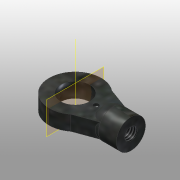
# Autodesk Inventor part: 500-103
Saved by Autodesk Inventor 2016 (Build 200138000, 138)
## iProperties
Created: 2015-04-18
Part Number: 500-103
Material: Steel
Document SubType Name: Modeling
Designer: Station9
Density: 7.85 g/cm^3
Appearance: Plate
Mass: 2.13897 g
Surface Area: 4.39252 cm^2
Volume: 0.27248 cm^3
Author: Station9
Autodesk Inventor part; units mm, degrees
ref_plane "YZ Plane" through (0, 0, 0) normal (1, 0, 0) x (0, 1, 0)
ref_plane "XZ Plane" through (0, 0, 0) normal (0, 1, 0) x (-1, 0, 0)
ref_plane "XY Plane" through (0, 0, 0) normal (0, 0, 1) x (1, 0, 0)
sketch "Sketch1" plane through (0, 0, 0) normal (0, 1, 0) x (-1, 0, 0)
  line L0 (3.5, 0) -> (-5.6696, 0) construction
  line L1 (0, -2.85) -> (3.5, -2.85)
  arc A0 (3.5, -2.85) -> (6.35, 0) centre (3.5, 0) ccw
  line L2 (0, 0) -> (0, -2.85)
  line L3 (0, 0) -> (6.35, 0)
  point P0 (-1.0848, 0)
  dimension "d0" = 2.85
  dimension "d1" = 3.5
  constraints: 10 end point, 2 point on circle, 1 centre point, 1 horizontal, 1 midpoint, 1 perpendicular, 1 tangent
  measures "d0" radius of A0
  measures "d1" distance from line of L2 L0.start
revolve "Revolution1" add sketch "Sketch1" angle 360 about axis through (-3.5, 0, 0) along (1, 0, 0)
sketch "Sketch2" plane through (0, 0, 0) normal (0, 0, 1) x (1, 0, 0)
  arc A0 (-7.7327, 3.9972) -> (-7.7396, -4.0028) centre (-10.9, 0) ccw
  line L0 (0, -2.85) -> (0, 2.85) projected
  line L1 (-3.5, -2.4597) -> (-7.7396, -4.0028)
  line L2 (-3.5, 2.4567) -> (-7.7327, 3.9972)
  arc A1 (-3.5, 2.85) -> (-6.35, 0) centre (-3.5, 0) ccw projected
  line L3 (-3.5, 2.85) -> (0, 2.85) projected
  line L4 (0, 2.85) -> (0, -2.85) projected
  line L5 (0, -2.85) -> (-3.5, -2.85) projected
  arc A2 (-6.35, 0) -> (-3.5, -2.85) centre (-3.5, 0) ccw projected
  line L6 (-3.5, 2.4567) -> (-3.5, -2.4597)
  line L7 (-3.5, -2.85) -> (-3.5, 2.85) projected
  point P0 (0, 0)
  dimension "d3" = 10.2
  dimension "d4" = 10.9
  dimension "d7" = 8
  dimension "d12" = 110
  dimension "d13" = 110
  constraints: 6 end point, 2 point on circle, 2 vertical alignment, 1 centre point, 1 collinear
  measures "d3" diameter of A0
  measures "d4" distance from line of L0 A0.centre
  measures "d7" distance of L1.end L2.end
  measures "d12" angle of L0 L2
  measures "d13" angle of L1 L6
extrude "Extrusion1" add sketch "Sketch2" along normal mid plane 2.9 contours L2 A1 A2 L1 A0 | L2 L6 L1 A2 A1
hole "Hole1" at (0, 0, 0) direction (-1, 0, 0) diameter 2.459 depth 6 tip angle 118 thread size "M3x0.5" class "6H" standard "ANSI Metric M Profile"
ref_plane "Work Plane1" through (-10.9, 0, 0) normal (1, 0, 0) x (0, 0, 1)
sketch "Sketch3" plane through (-10.9, 0, 0) normal (1, 0, 0) x (0, 0, 1)
  line L0 (-1.45, -5.1) -> (-1.45, 5.1) projected
  line L1 (-1.45, 5.1) -> (1.45, 5.1) projected
  line L2 (1.45, 5.1) -> (1.45, -5.1) projected
  line L3 (1.45, -5.1) -> (-1.45, -5.1) projected
  arc A0 (1.45, 2.8526) -> (-1.45, 2.8526) centre (0, 0) ccw
  line L4 (1.45, 0) -> (-1.45, 0)
  line L5 (-1.45, 2.8526) -> (-1.45, 0)
  line L6 (1.45, 0) -> (1.45, 2.8526)
  line L7 (-3.99, 0) -> (3.99, 0) projected
  constraints: 6 end point, 2 point on circle, 2 point on line, 1 centre point, 1 coincident, 1 midpoint
revolve "Revolution2" cut sketch "Sketch3" angle 360 about axis through (-10.9, 0, 0) along (0, 0, 1) contours L0 A0 L2 L4
sketch "Sketch4" plane through (0, 0, 1.45) normal (0, 0, 1) x (1, 0, 0)
  point P0 (0, 0)
  point P1 (-6.7959, 0)
hole "Hole2" at (-6.7959, 0, 1.45) direction (0, 0, -1) diameter 1 depth 0.5 tip angle 118
body "Solid1"
